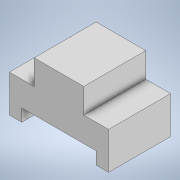
# Autodesk Inventor part: 7.1 Part 2
Saved by Autodesk Inventor 2020 (Build 240168000, 168)
## iProperties
Created: 2019-10-18
Part Number: 7.1 Part 2
Material: Generic
Document SubType Name: Modeling
Designer: cks4a449
Density: 1 g/cm^3
Appearance: Default
Author: cks4a449
Autodesk Inventor part; units mm, degrees
ref_plane "YZ Plane" through (0, 0, 0) normal (1, 0, 0) x (0, 1, 0)
ref_plane "XZ Plane" through (0, 0, 0) normal (0, 1, 0) x (-1, 0, 0)
ref_plane "XY Plane" through (0, 0, 0) normal (0, 0, 1) x (1, 0, 0)
sketch "Sketch2" plane through (0, 0, 0) normal (0, 0, 1) x (1, 0, 0)
  line L0 (0, 0) -> (25.4, 0)
  line L1 (25.4, 0) -> (25.4, 25.4)
  line L2 (25.4, 25.4) -> (177.8, 25.4)
  line L3 (177.8, 25.4) -> (177.8, 0)
  line L4 (177.8, 0) -> (203.2, 0)
  line L5 (203.2, 0) -> (203.2, 76.2)
  line L6 (203.2, 76.2) -> (152.4, 76.2)
  line L7 (152.4, 76.2) -> (152.4, 127)
  line L8 (152.4, 127) -> (50.8, 127)
  line L9 (50.8, 127) -> (50.8, 76.2)
  line L10 (50.8, 76.2) -> (0, 76.2)
  line L11 (0, 76.2) -> (0, 0)
  dimension "d1" = 25.4
  dimension "d2" = 25.4
  dimension "d3" = 152.4
  dimension "d4" = 25.4
  dimension "d5" = 25.4
  dimension "d6" = 76.2
  dimension "d7" = 50.8
  dimension "d8" = 50.8
  dimension "d9" = 101.6
  dimension "d10" = 50.8
  constraints: 24 end point, 7 perpendicular, 4 point on line, 1 horizontal
  measures "d1" distance of L0.start L0.end
  measures "d2" distance of L0.end L1.end
  measures "d3" distance of L1.end L2.end
  measures "d4" distance of L2.end L3.end
  measures "d5" distance of L3.end L4.end
  measures "d6" distance of L4.end L5.end
  measures "d7" distance of L5.end L6.end
  measures "d8" distance of L6.end L7.end
  measures "d9" distance of L7.end L8.end
  measures "d10" distance of L8.end L9.end
extrude "Extrusion1" add sketch "Sketch2" along normal blind 127
body "Solid1"
